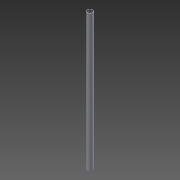
# Autodesk Inventor part: Belka
Saved by Autodesk Inventor 2015 (Build 190159000, 159)
## iProperties
Created: 2016-01-12
Part Number: Belka
Material: Aluminium AW-7020
Document SubType Name: Modeling
Designer: graaapsik
Density: 2.78 g/cm^3
Appearance: Aluminium AW-7020
Mass: 66.8123 g
Surface Area: 481.732 cm^2
Volume: 24.0332 cm^3
Author: graaapsik
Autodesk Inventor part; units mm, degrees
ref_plane "YZ Plane" through (0, 0, 0) normal (1, 0, 0) x (0, 1, 0)
ref_plane "XZ Plane" through (0, 0, 0) normal (0, 1, 0) x (-1, 0, 0)
ref_plane "XY Plane" through (0, 0, 0) normal (0, 0, 1) x (1, 0, 0)
sketch "Szkic1" plane through (0, 0, 0) normal (0, 0, 1) x (1, 0, 0)
  circle A0 centre (0, 0) radius 9
  dimension "d0" = 18
  constraints: 1 centre point, 1 coincident
  measures "d0" diameter of A0
extrude "Wyciągnięcie proste1" add sketch "Szkic1" along normal mid plane 450
shell "Skorupa1" thickness 1 removed faces 2 at (2.2455, -1.9894, 225) at (2.2455, -1.9894, -225)
thread "Gwint1" size "M16x2" class "6H" standard "ANSI Metric M Profile" length 15
thread "Gwint2" size "M16x2" class "6H" standard "ANSI Metric M Profile" length 15
